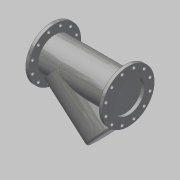
# Autodesk Inventor part: BALL CHECK VALVE FLANGED GGG50 DN250
Saved by Autodesk Inventor 2017 (Build 210142000, 142)
## iProperties
Category: Piping Part
Company: Demarec
Created: 2012-12-20
Part Number: BALL CHECK VALVE FLANGED GGG50 DN250
Material: GGG50
Document SubType Name: Modeling
Designer: Marc Crauwels
Density: 7.85 g/cm^3
Mass: 658107 g
Surface Area: 21375.3 cm^2
Volume: 83622.3 cm^3
Appearance: Steel
Catalog Web Link: http://www.pocketbrewery.com
Description: BV41
Author: Marc Crauwels
Title: Carbon Steel Globe Valve PN16
Comments: iPart CS GlbVlvPN16
Autodesk Inventor part; units mm, degrees
ref_plane "YZ Plane" through (0, 0, 0) normal (1, 0, 0) x (0, 1, 0)
ref_plane "XZ Plane" through (0, 0, 0) normal (0, 1, 0) x (-1, 0, 0)
ref_plane "XY Plane" through (0, 0, 0) normal (0, 0, 1) x (1, 0, 0)
sketch "Sketch1" plane through (0, 0, 0) normal (1, 0, 0) x (0, 1, 0)
  line L0 (274, 125) -> (298, 125)
  line L1 (298, 125) -> (298, 202.5)
  line L2 (298, 202.5) -> (274, 202.5)
  line L3 (274, 202.5) -> (274, 125)
  line L4 (298, 125) -> (300, 125)
  line L5 (300, 125) -> (300, 159)
  line L6 (300, 159) -> (298, 159)
  line L7 (298, 159) -> (298, 125)
  line L8 (-300, 0) -> (300, 0) construction
  line L9 (300, 0) -> (274, 0) construction
  line L10 (0, 0) -> (0, 224.4691) construction
  line L11 (-300, 0) -> (-274, 0) construction
  line L12 (0, 0) -> (-13.3333, 0)
  line L13 (0, -44.8938) -> (0, 269.363) projected
  dimension "Lenght" = 600
  dimension "DN" = 250
  dimension "FlgDia" = 405
  dimension "FlgThck" = 26
  dimension "GsktFace" = 318
  dimension "Face" = 2
  constraints: 26 end point, 5 point on line, 4 parallel, 3 horizontal, 3 perpendicular, 2 collinear, 1 coincident, 1 midpoint
  measures "Lenght" distance of L8.start L8.end
  measures "DN" diameter of L0 L8
  measures "FlgDia" diameter of L2 L8
  measures "FlgThck" distance between parallel lines of L3 L5
  measures "GsktFace" diameter of L5.end L8
  measures "Face" distance of L5.end L6.end
revolve "Revolution1" add sketch "Sketch1" angle 360 about axis through (0, -300, 0) along (0, 1, 0)
sketch "Sketch5" plane through (0, 298, 0) normal (0, 1, 0) x (1, 0, 0)
  line L0 (0, 0) -> (-45.9404, 171.4518)
  line L1 (0, 0) -> (0, 216.4053) construction
  circle A0 centre (-45.9404, 171.4518) radius 13.5
  dimension "d16" = 177.5
  dimension "d17" = 15
  dimension "d18" = 27
  constraints: 4 end point, 1 centre point, 1 coincident, 1 vertical
  measures "d16" distance of L0.start L0.end
  measures "d17" angle of L1 L0
  measures "d18" diameter of A0
extrude "Extrusion2" cut sketch "Sketch5" against normal through all
pattern_circular "Circular Pattern1" count 12 over 360 about axis through (0, 299, 0) along (0, 1, 0) of "Extrusion2"
sketch "Sketch14" plane through (0, 274, 0) normal (0, -1, 0) x (-1, 0, 0)
  circle A0 centre (0, 0) radius 125 projected
  circle A1 centre (0, 0) radius 131
  dimension "d54" = 6
  constraints: 1 centre point
  measures "d54" radial gap between concentric circles of A1 A0
pattern_circular "Circular Pattern2" count 2 over 360 about axis through (-10, 0, 0) along (1, 0, 0) of "Revolution1", "Extrusion2", "Circular Pattern1"
extrude "Extrusion5" add sketch "Sketch14" along normal up to surface (548 mm away) contours A0 | A1
sketch "Sketch21" plane through (0, 0, 0) normal (1, 0, 0) x (0, 1, 0)
  line L0 (-157.5433, -306.6743) -> (45.0425, -131)
  line L1 (-18.8207, 54.7375) -> (18.8207, -54.7375) construction
  line L2 (-157.5433, -306.6743) -> (-59.2718, -420)
  line L3 (-59.2718, -420) -> (274, -131)
  line L4 (274, -131) -> (45.0425, -131)
  line L5 (-157.5433, -306.6743) -> (-255.8148, -193.3486) construction
  line L6 (-255.8148, -193.3486) -> (-7.5443, 21.9416)
  line L7 (274, -131) -> (-274, -131) projected
  line L8 (-274, 202.5) -> (-274, -202.5) projected
  point P0 (0, 0)
  point P1 (0, 0)
  dimension "d79" = 150
  dimension "d86" = 5
  dimension "oH" = 420
  constraints: 14 end point, 4 perpendicular, 2 collinear, 2 point on line, 1 coincident, 1 midpoint
  measures "d79" distance of L0.start L2.end
  measures "d86" distance from line of L6 L8.end
  measures "oH" vertical distance of L2.end point (0, 0)
revolve "Revolution5" add sketch "Sketch21" angle 360 about axis through (0, -157.5433, -306.6743) along (0, 0.7555046, 0.6551434)
fillet "Fillet2" radius 15 1 edges at (0, -255.8148, -193.3486)
equation "\"d16\" = 0.5 * KDia"
equation "\"KDia\" = 355"
body "Solid1"
